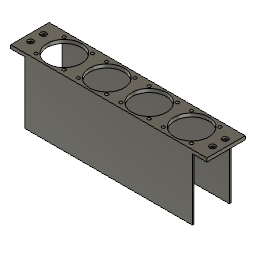
rear_fan_bar (Autodesk Fusion 360 design; units mm, degrees)
part number: 2026-08-22-19-03-56-576
Autodesk Fusion 360 part; units mm, degrees
sketch "Sketch1" plane through (0, 0, 0) normal (0, 0, 1) x (1, 0, 0)
  line L0 (-111, 0.4) -> (111, 0.4)
  line L1 (111, 0.4) -> (111, 44.05)
  line L2 (111, 44.05) -> (-111, 44.05)
  line L3 (-111, 44.05) -> (-111, 0.4)
extrude "Extrude1" add sketch "Sketch1" along normal blind 4
sketch "Sketch2" plane through (0, 0, 0) normal (0, 0, 1) x (1, 0, 0)
  circle A0 centre (-72, 22.225) radius 19.5
  circle A1 centre (-88, 6.225) radius 1.8
  circle A2 centre (-88, 38.225) radius 1.8
  circle A3 centre (-56, 6.225) radius 1.8
  circle A4 centre (-56, 38.225) radius 1.8
  circle A5 centre (-24, 22.225) radius 19.5
  circle A6 centre (-40, 6.225) radius 1.8
  circle A7 centre (-40, 38.225) radius 1.8
  circle A8 centre (-8, 6.225) radius 1.8
  circle A9 centre (-8, 38.225) radius 1.8
  circle A10 centre (24, 22.225) radius 19.5
  circle A11 centre (8, 6.225) radius 1.8
  circle A12 centre (8, 38.225) radius 1.8
  circle A13 centre (40, 6.225) radius 1.8
  circle A14 centre (40, 38.225) radius 1.8
  circle A15 centre (72, 22.225) radius 19.5
  circle A16 centre (56, 6.225) radius 1.8
  circle A17 centre (56, 38.225) radius 1.8
  circle A18 centre (88, 6.225) radius 1.8
  circle A19 centre (88, 38.225) radius 1.8
  circle A20 centre (-102.82, 15) radius 1.7
  circle A21 centre (-102.82, 29.45) radius 1.7
  circle A22 centre (102.82, 15) radius 1.7
  circle A23 centre (102.82, 29.45) radius 1.7
extrude "Extrude2" cut sketch "Sketch2" along normal blind 4
sketch "Sketch3" plane through (0, 0, 0) normal (0, 0, 1) x (1, 0, 0)
  line L0 (-94.8, 42.25) -> (94.8, 42.25)
  line L1 (94.8, 42.25) -> (94.8, 44.05)
  line L2 (94.8, 44.05) -> (-94.8, 44.05)
  line L3 (-94.8, 44.05) -> (-94.8, 42.25)
  line L4 (-94.8, 0.4) -> (94.8, 0.4)
  line L5 (94.8, 0.4) -> (94.8, 2.2)
  line L6 (94.8, 2.2) -> (-94.8, 2.2)
  line L7 (-94.8, 2.2) -> (-94.8, 0.4)
extrude "Extrude3" add sketch "Sketch3" against normal blind 70
ref_plane "WorkPlane1" through (0, 0, 4) normal (0, 0, 1) x (1, 0, 0)
sketch "Sketch4" plane through (0, 0, 4) normal (0, 0, 1) x (1, 0, 0)
  circle A0 centre (-102.82, 15) radius 3.25
  circle A1 centre (-102.82, 29.45) radius 3.25
  circle A2 centre (102.82, 15) radius 3.25
  circle A3 centre (102.82, 29.45) radius 3.25
extrude "Extrude4" cut sketch "Sketch4" against normal blind 2
named bodies: "Rear Fan Bar"
